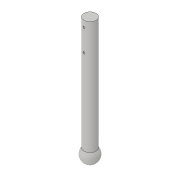
# Autodesk Inventor part: stik
Saved by Autodesk Inventor 2019 (Build 230136000, 136)
## iProperties
Created: 2020-02-15
Part Number: stik
Material: Generic
Document SubType Name: Modeling
Designer: Pranav naik
Density: 1 g/cm^3
Appearance: Default
Author: Pranav naik
Autodesk Inventor part; units mm, degrees
ref_plane "YZ Plane" through (0, 0, 0) normal (1, 0, 0) x (0, 1, 0)
ref_plane "XZ Plane" through (0, 0, 0) normal (0, 1, 0) x (-1, 0, 0)
ref_plane "XY Plane" through (0, 0, 0) normal (0, 0, 1) x (1, 0, 0)
sketch "Sketch1" plane through (0, 0, 0) normal (0, 0, 1) x (1, 0, 0)
  arc A0 (-7.5, 6.6144) -> (0, -10) centre (0, 0) ccw
  line L0 (0, 10) -> (0, -10)
  line L1 (-7.5, 6.6144) -> (0, 6.6144)
  dimension "d2" = 20
  constraints: 4 end point, 2 point on circle, 1 centre point, 1 horizontal, 1 point on line
  measures "d2" distance of L0.end L0.start
revolve "Revolution1" add sketch "Sketch1" angle 360 about axis through (0, 10, 0) along (0, -1, 0)
sketch "Sketch2" plane through (0, 6.6144, 0) normal (0, 1, 0) x (1, 0, 0)
  circle A0 centre (0, 0) radius 7.5
  constraints: 1 centre point, 1 coincident
extrude "Extrusion1" add sketch "Sketch2" along normal blind 140
sketch "Sketch3" plane through (0, 0, 0) normal (0, 0, 1) x (1, 0, 0)
  circle A0 centre (0, 111.8832) radius 1.25
  circle A1 centre (0, 139.0232) radius 1.25
  point P0 (0, 0)
  dimension "d8" = 2.5
  dimension "d9" = 2.5
  constraints: 2 centre point
  measures "d8" diameter of A0
  measures "d9" diameter of A1
extrude "Extrusion2" cut sketch "Sketch3" along normal mid plane 140
body "Solid1"
